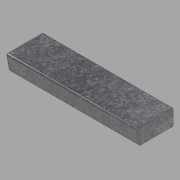
# Autodesk Inventor part: A
Saved by Autodesk Inventor 2022.1 (Build 261234020, 234B)
## iProperties
Created: 2021-12-14
Part Number: A
Material: Granite, Cut, Polished
Document SubType Name: Modeling
Designer: awelt
Density: 2.7 g/cm^3
Appearance: Kasota SN sapphire
Mass: 182552 g
Surface Area: 13789.3 cm^2
Volume: 67611.8 cm^3
Author: awelt
Autodesk Inventor part; units mm, degrees
ref_plane "YZ Plane" through (0, 0, 0) normal (1, 0, 0) x (0, 1, 0)
ref_plane "XZ Plane" through (0, 0, 0) normal (0, 1, 0) x (-1, 0, 0)
ref_plane "XY Plane" through (0, 0, 0) normal (0, 0, 1) x (1, 0, 0)
sketch "Sketch2" plane through (0, 0, 0) normal (1, 0, 0) x (0, 1, 0)
  line L0 (0, 0) -> (0, 152.4)
  line L1 (0, 0) -> (-330.2, 0)
  line L2 (0, 152.4) -> (-342.9, 152.4)
  line L3 (-342.9, 152.4) -> (-342.9, 139.7) construction
  arc A0 (-342.9, 152.4) -> (-355.3918, 137.4098) centre (-342.9, 139.7) ccw
  line L4 (-330.2, 0) -> (-355.3918, 137.4098)
  point P0 (355.6, 152.4)
  dimension "d0" = 152.4
  dimension "d14" = 342.9
  dimension "d15" = 330.2
  dimension "d16" = 12.7
  dimension "d17" = 139.7
  constraints: 10 end point, 2 point on circle, 2 vertical, 1 centre point, 1 coincident, 1 horizontal, 1 perpendicular, 1 tangent
  measures "d0" distance of L0.start L0.end
  measures "d14" distance of L0.end L2.end
  measures "d15" distance of L0.start L1.end
  measures "d16" distance of L2.end L3.end
  measures "d17" distance from line of L1 L3.end
extrude "Extrusion1" add sketch "Sketch2" along normal blind 1290.32
body "Solid1"
